Autodesk Inventor part; units mm, degrees
(part 15 of 15)
  line L1243 (16.475, -38.95) -> (17.125, -38.95)
  line L1244 (16.475, -37.25) -> (16.475, -37.682)
  line L1245 (17.325, -38.152) -> (17.325, -38.048)
  line L1246 (16.475, -38.518) -> (16.475, -38.95)
  line L1247 (17.125, -39.55) -> (16.475, -39.55)
  line L1248 (16.475, -41.25) -> (17.125, -41.25)
  line L1249 (16.475, -39.55) -> (16.475, -39.982)
  line L1250 (17.325, -40.452) -> (17.325, -40.348)
  line L1251 (16.475, -40.818) -> (16.475, -41.25)
  line L1252 (-12.6108, 53.143) -> (-17.5892, 53.143)
  line L1253 (-17.5892, 53.143) -> (-17.5892, 50.857)
  line L1254 (-17.5892, 50.857) -> (-12.6108, 50.857)
  line L1255 (-12.6108, 50.857) -> (-12.6108, 53.143)
  line L1256 (-8.4, -78.1) -> (-14.2, -78.1)
  line L1257 (-14.2, -78.1) -> (-14.2, -80.3)
  line L1258 (-14.2, -80.3) -> (-8.4, -80.3)
  line L1259 (-8.4, -80.3) -> (-8.4, -78.1)
  line L1260 (-22.657, -99.7892) -> (-22.657, -94.8108)
  line L1261 (-22.657, -94.8108) -> (-24.943, -94.8108)
  line L1262 (-24.943, -94.8108) -> (-24.943, -99.7892)
  line L1263 (-24.943, -99.7892) -> (-22.657, -99.7892)
  line L1264 (-20.057, -99.7892) -> (-20.057, -94.8108)
  line L1265 (-20.057, -94.8108) -> (-22.343, -94.8108)
  line L1266 (-22.343, -94.8108) -> (-22.343, -99.7892)
  line L1267 (-22.343, -99.7892) -> (-20.057, -99.7892)
  line L1268 (-13.616, 55.492) -> (-11.584, 55.492)
  line L1269 (-11.584, 55.492) -> (-11.584, 56.508)
  line L1270 (-11.584, 56.508) -> (-13.616, 56.508)
  line L1271 (-13.616, 56.508) -> (-13.616, 55.492)
  line L1272 (-11.584, 57.608) -> (-13.616, 57.608)
  line L1273 (-13.616, 57.608) -> (-13.616, 56.592)
  line L1274 (-13.616, 56.592) -> (-11.584, 56.592)
  line L1275 (-11.584, 56.592) -> (-11.584, 57.608)
  line L1276 (-15.792, 56.084) -> (-15.792, 58.116)
  line L1277 (-15.792, 58.116) -> (-16.808, 58.116)
  line L1278 (-16.808, 58.116) -> (-16.808, 56.084)
  line L1279 (-16.808, 56.084) -> (-15.792, 56.084)
  line L1280 (-20.584, -108.492) -> (-22.616, -108.492)
  line L1281 (-22.616, -108.492) -> (-22.616, -109.508)
  line L1282 (-22.616, -109.508) -> (-20.584, -109.508)
  line L1283 (-20.584, -109.508) -> (-20.584, -108.492)
  line L1284 (-13.784, -108.392) -> (-15.816, -108.392)
  line L1285 (-15.816, -108.392) -> (-15.816, -109.408)
  line L1286 (-15.816, -109.408) -> (-13.784, -109.408)
  line L1287 (-13.784, -109.408) -> (-13.784, -108.392)
  line L1288 (-20.584, -107.492) -> (-22.616, -107.492)
  line L1289 (-22.616, -107.492) -> (-22.616, -108.508)
  line L1290 (-22.616, -108.508) -> (-20.584, -108.508)
  line L1291 (-20.584, -108.508) -> (-20.584, -107.492)
  line L1292 (-13.784, -109.392) -> (-15.816, -109.392)
  line L1293 (-15.816, -109.392) -> (-15.816, -110.408)
  line L1294 (-15.816, -110.408) -> (-13.784, -110.408)
  line L1295 (-13.784, -110.408) -> (-13.784, -109.392)
  line L1296 (16.308, -112.816) -> (16.308, -110.784)
  line L1297 (16.308, -110.784) -> (15.292, -110.784)
  line L1298 (15.292, -110.784) -> (15.292, -112.816)
  line L1299 (15.292, -112.816) -> (16.308, -112.816)
  line L1300 (-9.684, -109.792) -> (-11.716, -109.792)
  line L1301 (-11.716, -109.792) -> (-11.716, -110.808)
  line L1302 (-11.716, -110.808) -> (-9.684, -110.808)
  line L1303 (-9.684, -110.808) -> (-9.684, -109.792)
  line L1304 (-2.884, -111.292) -> (-4.916, -111.292)
  line L1305 (-4.916, -111.292) -> (-4.916, -112.308)
  line L1306 (-4.916, -112.308) -> (-2.884, -112.308)
  line L1307 (-2.884, -112.308) -> (-2.884, -111.292)
  line L1308 (-4.908, -109.284) -> (-4.908, -111.316)
  line L1309 (-4.908, -111.316) -> (-3.892, -111.316)
  line L1310 (-3.892, -111.316) -> (-3.892, -109.284)
  line L1311 (-3.892, -109.284) -> (-4.908, -109.284)
  line L1312 (-4.908, -107.284) -> (-4.908, -109.316)
  line L1313 (-4.908, -109.316) -> (-3.892, -109.316)
  line L1314 (-3.892, -109.316) -> (-3.892, -107.284)
  line L1315 (-3.892, -107.284) -> (-4.908, -107.284)
  line L1316 (-9.484, 39.908) -> (-11.516, 39.908)
  line L1317 (-11.516, 39.908) -> (-11.516, 38.892)
  line L1318 (-11.516, 38.892) -> (-9.484, 38.892)
  line L1319 (-9.484, 38.892) -> (-9.484, 39.908)
  line L1320 (-9.484, 40.908) -> (-11.516, 40.908)
  line L1321 (-11.516, 40.908) -> (-11.516, 39.892)
  line L1322 (-11.516, 39.892) -> (-9.484, 39.892)
  line L1323 (-9.484, 39.892) -> (-9.484, 40.908)
  line L1324 (-0.392, -91.016) -> (-0.392, -88.984)
  line L1325 (-0.392, -88.984) -> (-1.408, -88.984)
  line L1326 (-1.408, -88.984) -> (-1.408, -91.016)
  line L1327 (-1.408, -91.016) -> (-0.392, -91.016)
  line L1328 (0.884, -93.508) -> (2.916, -93.508)
  line L1329 (2.916, -93.508) -> (2.916, -92.492)
  line L1330 (2.916, -92.492) -> (0.884, -92.492)
  line L1331 (0.884, -92.492) -> (0.884, -93.508)
  line L1332 (-1.116, -93.508) -> (0.916, -93.508)
  line L1333 (0.916, -93.508) -> (0.916, -92.492)
  line L1334 (0.916, -92.492) -> (-1.116, -92.492)
  line L1335 (-1.116, -92.492) -> (-1.116, -93.508)
  line L1336 (-21.584, -17.692) -> (-23.616, -17.692)
  line L1337 (-23.616, -17.692) -> (-23.616, -18.708)
  line L1338 (-23.616, -18.708) -> (-21.584, -18.708)
  line L1339 (-21.584, -18.708) -> (-21.584, -17.692)
  line L1340 (-23.616, -19.708) -> (-21.584, -19.708)
  line L1341 (-21.584, -19.708) -> (-21.584, -18.692)
  line L1342 (-21.584, -18.692) -> (-23.616, -18.692)
  line L1343 (-23.616, -18.692) -> (-23.616, -19.708)
  line L1344 (-19.584, -18.692) -> (-21.616, -18.692)
  line L1345 (-21.616, -18.692) -> (-21.616, -19.708)
  line L1346 (-21.616, -19.708) -> (-19.584, -19.708)
  line L1347 (-19.584, -19.708) -> (-19.584, -18.692)
  line L1348 (-19.584, -17.692) -> (-21.616, -17.692)
  line L1349 (-21.616, -17.692) -> (-21.616, -18.708)
  line L1350 (-21.616, -18.708) -> (-19.584, -18.708)
  line L1351 (-19.584, -18.708) -> (-19.584, -17.692)
  line L1352 (-19.584, -16.692) -> (-21.616, -16.692)
  line L1353 (-21.616, -16.692) -> (-21.616, -17.708)
  line L1354 (-21.616, -17.708) -> (-19.584, -17.708)
  line L1355 (-19.584, -17.708) -> (-19.584, -16.692)
  line L1356 (-24.608, -16.684) -> (-24.608, -18.716)
  line L1357 (-24.608, -18.716) -> (-23.592, -18.716)
  line L1358 (-23.592, -18.716) -> (-23.592, -16.684)
  line L1359 (-23.592, -16.684) -> (-24.608, -16.684)
  line L1360 (-19.816, -23.208) -> (-17.784, -23.208)
  line L1361 (-17.784, -23.208) -> (-17.784, -22.192)
  line L1362 (-17.784, -22.192) -> (-19.816, -22.192)
  line L1363 (-19.816, -22.192) -> (-19.816, -23.208)
  line L1364 (-21.816, -25.208) -> (-19.784, -25.208)
  line L1365 (-19.784, -25.208) -> (-19.784, -24.192)
  line L1366 (-19.784, -24.192) -> (-21.816, -24.192)
  line L1367 (-21.816, -24.192) -> (-21.816, -25.208)
  line L1368 (-21.816, -23.208) -> (-19.784, -23.208)
  line L1369 (-19.784, -23.208) -> (-19.784, -22.192)
  line L1370 (-19.784, -22.192) -> (-21.816, -22.192)
  line L1371 (-21.816, -22.192) -> (-21.816, -23.208)
  line L1372 (-17.816, -23.208) -> (-15.784, -23.208)
  line L1373 (-15.784, -23.208) -> (-15.784, -22.192)
  line L1374 (-15.784, -22.192) -> (-17.816, -22.192)
  line L1375 (-17.816, -22.192) -> (-17.816, -23.208)
  line L1376 (-16.708, -19.884) -> (-16.708, -21.916)
  line L1377 (-16.708, -21.916) -> (-15.692, -21.916)
  line L1378 (-15.692, -21.916) -> (-15.692, -19.884)
  line L1379 (-15.692, -19.884) -> (-16.708, -19.884)
  line L1380 (-14.292, -42.616) -> (-14.292, -40.584)
  line L1381 (-14.292, -40.584) -> (-15.308, -40.584)
  line L1382 (-15.308, -40.584) -> (-15.308, -42.616)
  line L1383 (-15.308, -42.616) -> (-14.292, -42.616)
  line L1384 (4.292, -38.784) -> (4.292, -40.816)
  line L1385 (4.292, -40.816) -> (5.308, -40.816)
  line L1386 (5.308, -40.816) -> (5.308, -38.784)
  line L1387 (5.308, -38.784) -> (4.292, -38.784)
  line L1388 (2.284, -41.408) -> (4.316, -41.408)
  line L1389 (4.316, -41.408) -> (4.316, -40.392)
  line L1390 (4.316, -40.392) -> (2.284, -40.392)
  line L1391 (2.284, -40.392) -> (2.284, -41.408)
  line L1392 (-15.292, -40.416) -> (-15.292, -38.384)
  line L1393 (-15.292, -38.384) -> (-16.308, -38.384)
  line L1394 (-16.308, -38.384) -> (-16.308, -40.416)
  line L1395 (-16.308, -40.416) -> (-15.292, -40.416)
  line L1396 (-16.308, -36.384) -> (-16.308, -38.416)
  line L1397 (-16.308, -38.416) -> (-15.292, -38.416)
  line L1398 (-15.292, -38.416) -> (-15.292, -36.384)
  line L1399 (-15.292, -36.384) -> (-16.308, -36.384)
  line L1400 (-11.3458, -38.111) -> (-15.0542, -38.111)
  line L1401 (-15.0542, -38.111) -> (-15.0542, -39.889)
  line L1402 (-15.0542, -39.889) -> (-11.3458, -39.889)
  line L1403 (-11.3458, -39.889) -> (-11.3458, -38.111)
  line L1404 (-15.0542, -38.089) -> (-11.3458, -38.089)
  line L1405 (-11.3458, -38.089) -> (-11.3458, -36.311)
  line L1406 (-11.3458, -36.311) -> (-15.0542, -36.311)
  line L1407 (-15.0542, -36.311) -> (-15.0542, -38.089)
  line L1408 (-4.092, -42.516) -> (-4.092, -40.484)
  line L1409 (-4.092, -40.484) -> (-5.108, -40.484)
  line L1410 (-5.108, -40.484) -> (-5.108, -42.516)
  line L1411 (-5.108, -42.516) -> (-4.092, -42.516)
  line L1412 (8.192, -38.784) -> (8.192, -40.816)
  line L1413 (8.192, -40.816) -> (9.208, -40.816)
  line L1414 (9.208, -40.816) -> (9.208, -38.784)
  line L1415 (9.208, -38.784) -> (8.192, -38.784)
  line L1416 (6.184, -41.408) -> (8.216, -41.408)
  line L1417 (8.216, -41.408) -> (8.216, -40.392)
  line L1418 (8.216, -40.392) -> (6.184, -40.392)
  line L1419 (6.184, -40.392) -> (6.184, -41.408)
  line L1420 (-8.384, -38.192) -> (-10.416, -38.192)
  line L1421 (-10.416, -38.192) -> (-10.416, -39.208)
  line L1422 (-10.416, -39.208) -> (-8.384, -39.208)
  line L1423 (-8.384, -39.208) -> (-8.384, -38.192)
  line L1424 (-8.384, -37.192) -> (-10.416, -37.192)
  line L1425 (-10.416, -37.192) -> (-10.416, -38.208)
  line L1426 (-10.416, -38.208) -> (-8.384, -38.208)
  line L1427 (-8.384, -38.208) -> (-8.384, -37.192)
  line L1428 (-3.7458, -38.111) -> (-7.4542, -38.111)
  line L1429 (-7.4542, -38.111) -> (-7.4542, -39.889)
  line L1430 (-7.4542, -39.889) -> (-3.7458, -39.889)
  line L1431 (-3.7458, -39.889) -> (-3.7458, -38.111)
  line L1432 (-7.4542, -38.089) -> (-3.7458, -38.089)
  line L1433 (-3.7458, -38.089) -> (-3.7458, -36.311)
  line L1434 (-3.7458, -36.311) -> (-7.4542, -36.311)
  line L1435 (-7.4542, -36.311) -> (-7.4542, -38.089)
  line L1436 (19.108, -39.116) -> (19.108, -37.084)
  line L1437 (19.108, -37.084) -> (18.092, -37.084)
  line L1438 (18.092, -37.084) -> (18.092, -39.116)
  line L1439 (18.092, -39.116) -> (19.108, -39.116)
  line L1440 (19.108, -41.416) -> (19.108, -39.384)
  line L1441 (19.108, -39.384) -> (18.092, -39.384)
  line L1442 (18.092, -39.384) -> (18.092, -41.416)
  line L1443 (18.092, -41.416) -> (19.108, -41.416)
  line L1444 (21.892, -41.484) -> (21.892, -43.516)
  line L1445 (21.892, -43.516) -> (22.908, -43.516)
  line L1446 (22.908, -43.516) -> (22.908, -41.484)
  line L1447 (22.908, -41.484) -> (21.892, -41.484)
  line L1448 (20.884, -41.508) -> (22.916, -41.508)
  line L1449 (22.916, -41.508) -> (22.916, -40.492)
  line L1450 (22.916, -40.492) -> (20.884, -40.492)
  line L1451 (20.884, -40.492) -> (20.884, -41.508)
  line L1452 (23.908, -43.516) -> (23.908, -41.484)
  line L1453 (23.908, -41.484) -> (22.892, -41.484)
  line L1454 (22.892, -41.484) -> (22.892, -43.516)
  line L1455 (22.892, -43.516) -> (23.908, -43.516)
  line L1456 (15.708, -39.916) -> (15.708, -37.884)
  line L1457 (15.708, -37.884) -> (14.692, -37.884)
  line L1458 (14.692, -37.884) -> (14.692, -39.916)
  line L1459 (14.692, -39.916) -> (15.708, -39.916)
  line L1460 (14.692, -39.984) -> (14.692, -42.016)
  line L1461 (14.692, -42.016) -> (15.708, -42.016)
  line L1462 (15.708, -42.016) -> (15.708, -39.984)
  line L1463 (15.708, -39.984) -> (14.692, -39.984)
  line L1464 (9.365, -39.203) -> (9.365, -41.997)
  line L1465 (9.365, -41.997) -> (10.635, -41.997)
  line L1466 (10.635, -41.997) -> (10.635, -39.203)
  line L1467 (10.635, -39.203) -> (9.365, -39.203)
  line L1468 (10.765, -39.203) -> (10.765, -41.997)
  line L1469 (10.765, -41.997) -> (12.035, -41.997)
  line L1470 (12.035, -41.997) -> (12.035, -39.203)
  line L1471 (12.035, -39.203) -> (10.765, -39.203)
  line L1472 (9.365, -42.203) -> (9.365, -44.997)
  line L1473 (9.365, -44.997) -> (10.635, -44.997)
  line L1474 (10.635, -44.997) -> (10.635, -42.203)
  line L1475 (10.635, -42.203) -> (9.365, -42.203)
  line L1476 (10.765, -42.203) -> (10.765, -44.997)
  line L1477 (10.765, -44.997) -> (12.035, -44.997)
  line L1478 (12.035, -44.997) -> (12.035, -42.203)
  line L1479 (12.035, -42.203) -> (10.765, -42.203)
  line L1480 (12.892, -37.884) -> (12.892, -39.916)
  line L1481 (12.892, -39.916) -> (13.908, -39.916)
  line L1482 (13.908, -39.916) -> (13.908, -37.884)
  line L1483 (13.908, -37.884) -> (12.892, -37.884)
  line L1484 (12.892, -39.984) -> (12.892, -42.016)
  line L1485 (12.892, -42.016) -> (13.908, -42.016)
  line L1486 (13.908, -42.016) -> (13.908, -39.984)
  line L1487 (13.908, -39.984) -> (12.892, -39.984)
  line L1488 (17.216, -45.192) -> (15.184, -45.192)
  line L1489 (15.184, -45.192) -> (15.184, -46.208)
  line L1490 (15.184, -46.208) -> (17.216, -46.208)
  line L1491 (17.216, -46.208) -> (17.216, -45.192)
  line L1492 (13.208, -47.216) -> (13.208, -45.184)
  line L1493 (13.208, -45.184) -> (12.192, -45.184)
  line L1494 (12.192, -45.184) -> (12.192, -47.216)
  line L1495 (12.192, -47.216) -> (13.208, -47.216)
  line L1496 (18.208, -47.216) -> (18.208, -45.184)
  line L1497 (18.208, -45.184) -> (17.192, -45.184)
  line L1498 (17.192, -45.184) -> (17.192, -47.216)
  line L1499 (17.192, -47.216) -> (18.208, -47.216)
  line L1500 (14.108, -50.316) -> (14.108, -48.284)
  line L1501 (14.108, -48.284) -> (13.092, -48.284)
  line L1502 (13.092, -48.284) -> (13.092, -50.316)
  line L1503 (13.092, -50.316) -> (14.108, -50.316)
  line L1504 (6.492, -42.484) -> (6.492, -44.516)
  line L1505 (6.492, -44.516) -> (7.508, -44.516)
  line L1506 (7.508, -44.516) -> (7.508, -42.484)
  line L1507 (7.508, -42.484) -> (6.492, -42.484)
  line L1508 (10.284, -51.808) -> (12.316, -51.808)
  line L1509 (12.316, -51.808) -> (12.316, -50.792)
  line L1510 (12.316, -50.792) -> (10.284, -50.792)
  line L1511 (10.284, -50.792) -> (10.284, -51.808)
  line L1512 (12.316, -51.792) -> (10.284, -51.792)
  line L1513 (10.284, -51.792) -> (10.284, -52.808)
  line L1514 (10.284, -52.808) -> (12.316, -52.808)
  line L1515 (12.316, -52.808) -> (12.316, -51.792)
  line L1516 (11.308, -50.816) -> (11.308, -48.784)
  line L1517 (11.308, -48.784) -> (10.292, -48.784)
  line L1518 (10.292, -48.784) -> (10.292, -50.816)
  line L1519 (10.292, -50.816) -> (11.308, -50.816)
  line L1520 (11.292, -48.784) -> (11.292, -50.816)
  line L1521 (11.292, -50.816) -> (12.308, -50.816)
  line L1522 (12.308, -50.816) -> (12.308, -48.784)
  line L1523 (12.308, -48.784) -> (11.292, -48.784)
  line L1524 (10.992, -54.784) -> (10.992, -56.816)
  line L1525 (10.992, -56.816) -> (12.008, -56.816)
  line L1526 (12.008, -56.816) -> (12.008, -54.784)
  line L1527 (12.008, -54.784) -> (10.992, -54.784)
  line L1528 (11.008, -56.816) -> (11.008, -54.784)
  line L1529 (11.008, -54.784) -> (9.992, -54.784)
  line L1530 (9.992, -54.784) -> (9.992, -56.816)
  line L1531 (9.992, -56.816) -> (11.008, -56.816)
  line L1532 (3.992, -54.784) -> (3.992, -56.816)
  line L1533 (3.992, -56.816) -> (5.008, -56.816)
  line L1534 (5.008, -56.816) -> (5.008, -54.784)
  line L1535 (5.008, -54.784) -> (3.992, -54.784)
  line L1536 (2.992, -54.784) -> (2.992, -56.816)
  line L1537 (2.992, -56.816) -> (4.008, -56.816)
  line L1538 (4.008, -56.816) -> (4.008, -54.784)
  line L1539 (4.008, -54.784) -> (2.992, -54.784)
  line L1540 (1.708, -44.516) -> (1.708, -42.484)
  line L1541 (1.708, -42.484) -> (0.692, -42.484)
  line L1542 (0.692, -42.484) -> (0.692, -44.516)
  line L1543 (0.692, -44.516) -> (1.708, -44.516)
  line L1544 (6.508, -44.516) -> (6.508, -42.484)
  line L1545 (6.508, -42.484) -> (5.492, -42.484)
  line L1546 (5.492, -42.484) -> (5.492, -44.516)
  line L1547 (5.492, -44.516) -> (6.508, -44.516)
  line L1548 (-16.284, -42.692) -> (-18.316, -42.692)
  line L1549 (-18.316, -42.692) -> (-18.316, -43.708)
  line L1550 (-18.316, -43.708) -> (-16.284, -43.708)
  line L1551 (-16.284, -43.708) -> (-16.284, -42.692)
  line L1552 (-16.284, -45.692) -> (-18.316, -45.692)
  line L1553 (-18.316, -45.692) -> (-18.316, -46.708)
  line L1554 (-18.316, -46.708) -> (-16.284, -46.708)
  line L1555 (-16.284, -46.708) -> (-16.284, -45.692)
  line L1556 (-16.284, -48.692) -> (-18.316, -48.692)
  line L1557 (-18.316, -48.692) -> (-18.316, -49.708)
  line L1558 (-18.316, -49.708) -> (-16.284, -49.708)
  line L1559 (-16.284, -49.708) -> (-16.284, -48.692)
  line L1560 (-16.284, -51.592) -> (-18.316, -51.592)
  line L1561 (-18.316, -51.592) -> (-18.316, -52.608)
  line L1562 (-18.316, -52.608) -> (-16.284, -52.608)
  line L1563 (-16.284, -52.608) -> (-16.284, -51.592)
  line L1564 (7.992, -54.784) -> (7.992, -56.816)
  line L1565 (7.992, -56.816) -> (9.008, -56.816)
  line L1566 (9.008, -56.816) -> (9.008, -54.784)
  line L1567 (9.008, -54.784) -> (7.992, -54.784)
  line L1568 (10.008, -56.816) -> (10.008, -54.784)
  line L1569 (10.008, -54.784) -> (8.992, -54.784)
  line L1570 (8.992, -54.784) -> (8.992, -56.816)
  line L1571 (8.992, -56.816) -> (10.008, -56.816)
  line L1572 (6.992, -54.784) -> (6.992, -56.816)
  line L1573 (6.992, -56.816) -> (8.008, -56.816)
  line L1574 (8.008, -56.816) -> (8.008, -54.784)
  line L1575 (8.008, -54.784) -> (6.992, -54.784)
  line L1576 (7.008, -56.816) -> (7.008, -54.784)
  line L1577 (7.008, -54.784) -> (5.992, -54.784)
  line L1578 (5.992, -54.784) -> (5.992, -56.816)
  line L1579 (5.992, -56.816) -> (7.008, -56.816)
  line L1580 (-1.016, -55.808) -> (1.016, -55.808)
  line L1581 (1.016, -55.808) -> (1.016, -54.792)
  line L1582 (1.016, -54.792) -> (-1.016, -54.792)
  line L1583 (-1.016, -54.792) -> (-1.016, -55.808)
  line L1584 (-3.016, -55.808) -> (-0.984, -55.808)
  line L1585 (-0.984, -55.808) -> (-0.984, -54.792)
  line L1586 (-0.984, -54.792) -> (-3.016, -54.792)
  line L1587 (-3.016, -54.792) -> (-3.016, -55.808)
  line L1588 (-1.016, -56.808) -> (1.016, -56.808)
  line L1589 (1.016, -56.808) -> (1.016, -55.792)
  line L1590 (1.016, -55.792) -> (-1.016, -55.792)
  line L1591 (-1.016, -55.792) -> (-1.016, -56.808)
  line L1592 (-3.016, -56.808) -> (-0.984, -56.808)
  line L1593 (-0.984, -56.808) -> (-0.984, -55.792)
  line L1594 (-0.984, -55.792) -> (-3.016, -55.792)
  line L1595 (-3.016, -55.792) -> (-3.016, -56.808)
  line L1596 (0.992, -54.784) -> (0.992, -56.816)
  line L1597 (0.992, -56.816) -> (2.008, -56.816)
  line L1598 (2.008, -56.816) -> (2.008, -54.784)
  line L1599 (2.008, -54.784) -> (0.992, -54.784)
  line L1600 (3.008, -56.816) -> (3.008, -54.784)
  line L1601 (3.008, -54.784) -> (1.992, -54.784)
  line L1602 (1.992, -54.784) -> (1.992, -56.816)
  line L1603 (1.992, -56.816) -> (3.008, -56.816)
  line L1604 (9.616, 52.008) -> (7.584, 52.008)
  line L1605 (7.584, 52.008) -> (7.584, 50.992)
  line L1606 (7.584, 50.992) -> (9.616, 50.992)
  line L1607 (9.616, 50.992) -> (9.616, 52.008)
  line L1608 (9.616, 53.008) -> (7.584, 53.008)
  line L1609 (7.584, 53.008) -> (7.584, 51.992)
  line L1610 (7.584, 51.992) -> (9.616, 51.992)
  line L1611 (9.616, 51.992) -> (9.616, 53.008)
  line L1612 (9.616, 54.008) -> (7.584, 54.008)
  line L1613 (7.584, 54.008) -> (7.584, 52.992)
  line L1614 (7.584, 52.992) -> (9.616, 52.992)
  line L1615 (9.616, 52.992) -> (9.616, 54.008)
  line L1616 (9.616, 55.008) -> (7.584, 55.008)
  line L1617 (7.584, 55.008) -> (7.584, 53.992)
  line L1618 (7.584, 53.992) -> (9.616, 53.992)
  line L1619 (9.616, 53.992) -> (9.616, 55.008)
  circle A188 centre (-47.2, -40.002) radius 0.65
  circle A189 centre (-47.2, -40.002) radius 0.65
  circle A190 centre (-45.449, -40.417) radius 0.65
  circle A191 centre (-45.449, -40.417) radius 0.65
  circle A192 centre (-43.841, -41.225) radius 0.65
  circle A193 centre (-43.841, -41.225) radius 0.65
  circle A194 centre (-42.463, -42.382) radius 0.65
  circle A195 centre (-42.463, -42.382) radius 0.65
  circle A196 centre (-41.388, -43.825) radius 0.65
  circle A197 centre (-41.388, -43.825) radius 0.65
  circle A198 centre (-40.676, -45.477) radius 0.65
  circle A199 centre (-40.676, -45.477) radius 0.65
  circle A200 centre (-40.363, -47.249) radius 0.65
  circle A201 centre (-40.363, -47.249) radius 0.65
  circle A202 centre (-40.468, -49.046) radius 0.65
  circle A203 centre (-40.468, -49.046) radius 0.65
  circle A204 centre (-40.984, -50.77) radius 0.65
  circle A205 centre (-40.984, -50.77) radius 0.65
  circle A206 centre (-41.884, -52.328) radius 0.65
  circle A207 centre (-41.884, -52.328) radius 0.65
  circle A208 centre (-43.118, -53.637) radius 0.65
  circle A209 centre (-43.118, -53.637) radius 0.65
  circle A210 centre (-44.622, -54.626) radius 0.65
  circle A211 centre (-44.622, -54.626) radius 0.65
  circle A212 centre (-46.313, -55.241) radius 0.65
  circle A213 centre (-46.313, -55.241) radius 0.65
  circle A214 centre (-48.1, -55.45) radius 0.65
  circle A215 centre (-48.1, -55.45) radius 0.65
  circle A216 centre (-49.887, -55.241) radius 0.65
  circle A217 centre (-49.887, -55.241) radius 0.65
  circle A218 centre (-51.578, -54.626) radius 0.65
  circle A219 centre (-51.578, -54.626) radius 0.65
  circle A220 centre (-53.082, -53.637) radius 0.65
  circle A221 centre (-53.082, -53.637) radius 0.65
  circle A222 centre (-54.316, -52.328) radius 0.65
  circle A223 centre (-54.316, -52.328) radius 0.65
  circle A224 centre (-55.216, -50.77) radius 0.65
  circle A225 centre (-55.216, -50.77) radius 0.65
  circle A226 centre (-55.732, -49.046) radius 0.65
  circle A227 centre (-55.732, -49.046) radius 0.65
  circle A228 centre (-55.837, -47.249) radius 0.65
  circle A229 centre (-55.837, -47.249) radius 0.65
  circle A230 centre (-55.524, -45.477) radius 0.65
  circle A231 centre (-55.524, -45.477) radius 0.65
  circle A232 centre (-54.812, -43.825) radius 0.65
  circle A233 centre (-54.812, -43.825) radius 0.65
  circle A234 centre (-53.737, -42.382) radius 0.65
  circle A235 centre (-53.737, -42.382) radius 0.65
  circle A236 centre (-52.359, -41.225) radius 0.65
  circle A237 centre (-52.359, -41.225) radius 0.65
  circle A238 centre (-50.751, -40.417) radius 0.65
  circle A239 centre (-50.751, -40.417) radius 0.65
  circle A240 centre (-49, -40.002) radius 0.65
  circle A241 centre (-49, -40.002) radius 0.65
  circle A242 centre (-47.181, -41.897) radius 0.65
  circle A243 centre (-47.181, -41.897) radius 0.65
  circle A244 centre (-45.433, -42.465) radius 0.65
  circle A245 centre (-45.433, -42.465) radius 0.65
  circle A246 centre (-43.946, -43.546) radius 0.65
  circle A247 centre (-43.946, -43.546) radius 0.65
  circle A248 centre (-42.865, -45.033) radius 0.65
  circle A249 centre (-42.865, -45.033) radius 0.65
  circle A250 centre (-42.297, -46.781) radius 0.65
  circle A251 centre (-42.297, -46.781) radius 0.65
  circle A252 centre (-42.297, -48.619) radius 0.65
  circle A253 centre (-42.297, -48.619) radius 0.65
  circle A254 centre (-42.865, -50.367) radius 0.65
  circle A255 centre (-42.865, -50.367) radius 0.65
  circle A256 centre (-43.946, -51.854) radius 0.65
  circle A257 centre (-43.946, -51.854) radius 0.65
  circle A258 centre (-45.433, -52.935) radius 0.65
  circle A259 centre (-45.433, -52.935) radius 0.65
  circle A260 centre (-47.181, -53.503) radius 0.65
  circle A261 centre (-47.181, -53.503) radius 0.65
  circle A262 centre (-49.019, -53.503) radius 0.65
  circle A263 centre (-49.019, -53.503) radius 0.65
  circle A264 centre (-50.767, -52.935) radius 0.65
  circle A265 centre (-50.767, -52.935) radius 0.65
  circle A266 centre (-52.254, -51.854) radius 0.65
  circle A267 centre (-52.254, -51.854) radius 0.65
  circle A268 centre (-53.335, -50.367) radius 0.65
  circle A269 centre (-53.335, -50.367) radius 0.65
  circle A270 centre (-53.903, -48.619) radius 0.65
  circle A271 centre (-53.903, -48.619) radius 0.65
  circle A272 centre (-53.903, -46.781) radius 0.65
  circle A273 centre (-53.903, -46.781) radius 0.65
  circle A274 centre (-53.335, -45.033) radius 0.65
  circle A275 centre (-53.335, -45.033) radius 0.65
  circle A276 centre (-52.254, -43.546) radius 0.65
  circle A277 centre (-52.254, -43.546) radius 0.65
  circle A278 centre (-50.767, -42.465) radius 0.65
  circle A279 centre (-50.767, -42.465) radius 0.65
  circle A280 centre (-49.019, -41.897) radius 0.65
  circle A281 centre (-49.019, -41.897) radius 0.65
  circle A282 centre (-47.143, -43.816) radius 0.65
  circle A283 centre (-47.143, -43.816) radius 0.65
  circle A284 centre (-45.448, -44.706) radius 0.65
  circle A285 centre (-45.448, -44.706) radius 0.65
  circle A286 centre (-44.36, -46.282) radius 0.65
  circle A287 centre (-44.36, -46.282) radius 0.65
  circle A288 centre (-44.129, -48.182) radius 0.65
  circle A289 centre (-44.129, -48.182) radius 0.65
  circle A290 centre (-44.808, -49.972) radius 0.65
  circle A291 centre (-44.808, -49.972) radius 0.65
  circle A292 centre (-46.241, -51.242) radius 0.65
  circle A293 centre (-46.241, -51.242) radius 0.65
  circle A294 centre (-48.1, -51.7) radius 0.65
  circle A295 centre (-48.1, -51.7) radius 0.65
  circle A296 centre (-49.959, -51.242) radius 0.65
  circle A297 centre (-49.959, -51.242) radius 0.65
  circle A298 centre (-51.392, -49.972) radius 0.65
  circle A299 centre (-51.392, -49.972) radius 0.65
  circle A300 centre (-52.071, -48.182) radius 0.65
  circle A301 centre (-52.071, -48.182) radius 0.65
  circle A302 centre (-51.84, -46.282) radius 0.65
  circle A303 centre (-51.84, -46.282) radius 0.65
  circle A304 centre (-50.752, -44.706) radius 0.65
  circle A305 centre (-50.752, -44.706) radius 0.65
  circle A306 centre (-49.057, -43.816) radius 0.65
  circle A307 centre (-49.057, -43.816) radius 0.65
  circle A308 centre (-48.1, -45.575) radius 0.65
  circle A309 centre (-48.1, -45.575) radius 0.65
  circle A310 centre (-46.439, -46.375) radius 0.65
  circle A311 centre (-46.439, -46.375) radius 0.65
  circle A312 centre (-46.028, -48.173) radius 0.65
  circle A313 centre (-46.028, -48.173) radius 0.65
  circle A314 centre (-47.178, -49.615) radius 0.65
  circle A315 centre (-47.178, -49.615) radius 0.65
  circle A316 centre (-49.022, -49.615) radius 0.65
  circle A317 centre (-49.022, -49.615) radius 0.65
  circle A318 centre (-50.172, -48.173) radius 0.65
  circle A319 centre (-50.172, -48.173) radius 0.65
  circle A320 centre (-49.761, -46.375) radius 0.65
  circle A321 centre (-49.761, -46.375) radius 0.65
  circle A322 centre (-48.1, -47.7) radius 0.65
  circle A323 centre (-48.1, -47.7) radius 0.65
  circle A324 centre (-39.845, -55.955) radius 0.75
  circle A325 centre (-39.845, -55.955) radius 0.75
  circle A326 centre (-56.355, -55.955) radius 0.75
  circle A327 centre (-56.355, -55.955) radius 0.75
  circle A328 centre (-56.355, -39.445) radius 0.75
  circle A329 centre (-56.355, -39.445) radius 0.75
  circle A330 centre (-39.845, -39.445) radius 0.75
  circle A331 centre (-39.845, -39.445) radius 0.75
  circle A332 centre (-25.982, 58.14) radius 1.0532
  circle A333 centre (-25.982, 58.14) radius 1.0532
  circle A334 centre (-20.902, 58.14) radius 1.0532
  circle A335 centre (-20.902, 58.14) radius 1.0532
  circle A336 centre (-20.902, 53.06) radius 1.0532
  circle A337 centre (-20.902, 53.06) radius 1.0532
  circle A338 centre (-25.982, 53.06) radius 1.0532
  circle A339 centre (-25.982, 53.06) radius 1.0532
  circle A340 centre (-23.442, 55.6) radius 0.9532
  circle A341 centre (-23.442, 55.6) radius 0.9532
  point P0 (0, 0)
  point P1 (-46.08, -39.482)
  point P2 (-44.329, -39.897)
  point P3 (-42.721, -40.705)
  point P4 (-41.343, -41.862)
  point P5 (-40.268, -43.305)
  point P6 (-39.556, -44.957)
  point P7 (-39.243, -46.729)
  point P8 (-39.348, -50.366)
  point P9 (-39.864, -52.09)
  point P10 (-40.114, -53.648)
  point P11 (-41.348, -54.957)
  point P12 (-42.852, -55.946)
  point P13 (-44.543, -56.561)
  point P14 (-48.62, -56.77)
  point P15 (-50.407, -56.561)
  point P16 (-52.098, -55.946)
  point P17 (-53.602, -54.957)
  point P18 (-54.836, -53.648)
  point P19 (-55.736, -52.09)
  point P20 (-56.252, -50.366)
  point P21 (-56.357, -46.729)
  point P22 (-56.044, -44.957)
  point P23 (-55.332, -43.305)
  point P24 (-54.257, -41.862)
  point P25 (-52.879, -40.705)
  point P26 (-51.271, -39.897)
  point P27 (-49.52, -39.482)
  point P28 (-22, 24.2)
  point P29 (11, 24.2)
  point P30 (-24, 21.2)
  point P31 (-24, -11.8)
  point P32 (13.6, 23)
  point P33 (25.3, 23.1)
  point P34 (12, 20.5)
  point P35 (12, 13.9)
  point P36 (13.6, 12.6)
  point P37 (25.3, 12.7)
  point P38 (12, 10.1)
  point P39 (12, 3.5)
  point P40 (13.6, 2.2)
  point P41 (25.3, 2.3)
  point P42 (12, -0.3)
  point P43 (12, -6.9)
  point P44 (13.6, -8.2)
  point P45 (25.3, -8.1)
  point P46 (12, -10.7)
  point P47 (12, -17.3)
  point P48 (10.2, -25.6)
  point P49 (-1.5, -25.7)
  point P50 (11.8, -23.1)
  point P51 (11.8, -16.5)
  point P52 (62.15, 52.6)
  point P53 (64.15, 50.6)
  point P54 (64.15, 38.6)
  point P55 (50.15, 52.6)
  point P56 (-20.9, -78.4)
  point P57 (-20.9, -84.9)
  point P58 (-20.9, -91.1)
  point P59 (-18.6, -97.3)
  point P60 (-11, -97.3)
  point P61 (-1, -107.6)
  point P62 (-1, -104.5)
  point P63 (-17.2, -105.2)
  point P64 (-17.2, -102)
  point P65 (-13.1, -108.8)
  point P66 (-14.8, -107.9)
  point P67 (-19.8, -111.3)
  point P68 (-15.7, -114.7)
  point P69 (18.6, -83.7)
  point P70 (11.3, -89.2)
  point P71 (18.6, -81.7)
  point P72 (14.4, -76.6)
  point P73 (5.2, -83.7)
  point P74 (15.8, -76.6)
  point P75 (8.8, -76.6)
  point P76 (5.2, -81.7)
  point P77 (13, -76.6)
  point P78 (11.6, -76.6)
  point P79 (9.1, -89.2)
  point P80 (7.1, -89.2)
  point P81 (5.3, -89.7)
  point P82 (10.2, -76.6)
  point P83 (18.6, -90.5)
  point P84 (-1.6, -85.3)
  point P85 (14.7, -91.6)
  point P86 (1.5, -85.3)
  point P87 (18.7, -96)
  point P88 (14.7, -94.6)
  point P89 (-1.2, -53.2)
  point P90 (18.4, -43)
  point P91 (1.4, -53.2)
  point P92 (23.1, -78.9)
  point P93 (23.1, -75.8)
  point P94 (-5, -77.5)
  point P95 (-5, -82.2)
  point P96 (1.2, -77.5)
  point P97 (-24.6, -20.3)
  point P98 (-1.9, -77.5)
  point P99 (23.1, -86.5)
  point P100 (23.1, -89.6)
  point P101 (23.1, -92.6)
  point P102 (23.1, -95.6)
  point P103 (15.8, -115.3)
  point P104 (11.2, -109)
  point P105 (2.6, -109.9)
  point P106 (4.4, -109.9)
  point P107 (9.4, -109.9)
  point P108 (10.3, -113.9)
  point P109 (5.3, -103.3)
  point P110 (17.8, -99)
  point P111 (9.4, -102.3)
  point P112 (7.8, -102.3)
  point P113 (-9.8, -106.1)
  point P114 (-10.8, -108.6)
  point P115 (-3.9, -112.8)
  point P116 (12.2, -97.6)
  point P117 (-8.8, -112.2)
  point P118 (18.4, -101.2)
  point P119 (17.1, -101.2)
  point P120 (-3.4, -110.3)
  point P121 (-11.2, -115.5)
  point P122 (5.3, -97.1)
  point P123 (-6.1, 46.4)
  point P124 (-6.8, 37.9)
  point P125 (-3.2, 41.2)
  point P126 (-5.6, 44.8)
  point P127 (-1.7, 44.6)
  point P128 (-3.2, 36.8)
  point P129 (-2.7, 47.4)
  point P130 (1.9, -94)
  point P131 (-24.6, -19.2)
  point P132 (-24.6, -16.2)
  point P133 (-25.1, -17.7)
  point P134 (-20.8, -25.7)
  point P135 (-23.2, -22.9)
  point P136 (-21.3, -21)
  point P137 (-2.8, -16.6)
  point P138 (-6.2, -21.6)
  point P139 (-2.8, -15.6)
  point P140 (-6.2, -19.6)
  point P141 (-6.2, -18.6)
  point P142 (-6.2, -16.6)
  point P143 (-2.8, -18.6)
  point P144 (-6.2, -15.6)
  point P145 (-6.2, -22.6)
  point P146 (-2.8, -21.6)
  point P147 (-2.8, -22.6)
  point P148 (-2.8, -19.6)
  point P149 (-6.2, -23.6)
  point P150 (1.8, -39.8)
  point P151 (3.3, -38.3)
  point P152 (-13.3, -41.1)
  point P153 (5.7, -39.8)
  point P154 (7.2, -38.3)
  point P155 (-5.6, -41.5)
  point P156 (21.4, -42.5)
  point P157 (14.2, -45.7)
  point P158 (14.6, -49.3)
  point P159 (17.3, -49.3)
  point P160 (14.2, -46.7)
  point P161 (16.2, -46.7)
  point P162 (5.5, -55.8)
  point P163 (-4.1, -52.2)
  point P164 (-4.1, -49.2)
  point P165 (-4.1, -46.2)
  point P166 (-4.1, -43.2)
  point P167 (6.4, 53)
  point P168 (6.4, 54)
  point P169 (-1.7, 59.2)
  point P170 (6, 55.2)
  point P171 (0.7, 58.3)
  point P172 (0.6, 53.8)
  point P173 (0.6, 52.8)
  point P174 (1, 51.6)
  point P175 (0.6, 57.2)
  point P176 (0.6, 56.2)
  point P177 (1, 55)
  point P178 (6.4, 51)
  point P179 (-1.6, 54.2)
  point P180 (-1.6, 56.2)
  point P181 (6.4, 52)
  point P182 (-1.6, 53.2)
  point P183 (-1.6, 55.2)
  point P184 (5.6, 35.1)
  point P185 (9.6, 43.5)
  point P186 (9.6, 42.5)
  point P187 (1.8, 42.8)
  point P188 (1.8, 40.8)
  point P189 (7.1, 47)
  point P190 (5.95, 47.4)
  point P191 (4.8, 47)
  point P192 (3.8, 47)
  point P193 (6.1, 36.6)
  point P194 (5.1, 36.6)
  point P195 (5.1, 38.6)
  point P196 (3.3, 43.3)
  point P197 (5.1, 45)
  point P198 (6.1, 38.6)
  point P199 (3.3, 42.3)
  constraints: 3240 end point, 341 centre point, 236 point on circle, 55 other
